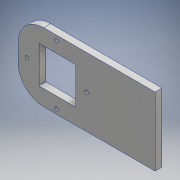
# Autodesk Inventor part: sholder_1
Saved by Autodesk Inventor 2016 (Build 200138000, 138)
## iProperties
Created: 2016-06-28
Part Number: sholder_1
Material: アルミニウム 6061
Document SubType Name: Modeling
Designer: 宏太
Density: 2.7 g/cm^3
Appearance: アルミニウム - フラット
Mass: 227.001 g
Surface Area: 264.508 cm^2
Volume: 84.0744 cm^3
Author: 宏太
Autodesk Inventor part; units mm, degrees
ref_plane "YZ Plane" through (0, 0, 0) normal (1, 0, 0) x (0, 1, 0)
ref_plane "XZ Plane" through (0, 0, 0) normal (0, 1, 0) x (-1, 0, 0)
ref_plane "XY Plane" through (0, 0, 0) normal (0, 0, 1) x (1, 0, 0)
sketch "スケッチ1" plane through (0, 0, 0) normal (0, 1, 0) x (-1, 0, 0)
  line L0 (-80, -40) -> (80, -40)
  line L1 (80, -40) -> (80, 40)
  line L2 (80, 40) -> (-80, 40)
  line L3 (-80, 40) -> (-80, -40)
  line L4 (-80, -40) -> (80, 40) construction
  line L5 (80, -40) -> (-80, 40) construction
  point P0 (0, 0)
  dimension "d0" = 160
  dimension "d1" = 80
  constraints: 12 end point, 2 midpoint, 2 parallel, 1 horizontal, 1 perpendicular
  measures "d0" distance of L2.end L1.end
  measures "d1" distance of L1.end L0.end
extrude "押し出し1" add sketch "スケッチ1" along normal blind 8
sketch "スケッチ2" plane through (0, 8, 0) normal (0, 1, 0) x (1, 0, 0)
  line L0 (-12.5, 21.5) -> (-55.5, 21.5)
  line L1 (-55.5, 21.5) -> (-55.5, -21.5)
  line L2 (-55.5, -21.5) -> (-12.5, -21.5)
  line L3 (-12.5, -21.5) -> (-12.5, 21.5)
  line L4 (-12.5, 21.5) -> (-55.5, -21.5) construction
  line L5 (-55.5, 21.5) -> (-12.5, -21.5) construction
  line L6 (-80, 40) -> (-80, -40) projected
  line L7 (-80, -40) -> (80, -40) projected
  point P0 (0, 0)
  point P1 (-34, 0)
  dimension "d4" = 43
  dimension "d5" = 43
  dimension "d20" = 46
  dimension "d21" = 40
  constraints: 12 end point, 2 midpoint, 2 parallel, 1 horizontal, 1 perpendicular
  measures "d4" distance of L2.end L1.end
  measures "d5" distance of L1.end L0.end
  measures "d20" distance from line of L6 point (-34, 0)
  measures "d21" distance from line of L7 point (-34, 0)
extrude "押し出し2" cut sketch "スケッチ2" against normal blind 8
sketch "スケッチ3" plane through (0, 8, 0) normal (0, 1, 0) x (1, 0, 0)
  circle A0 centre (-35, 0) radius 34.5
  circle A1 centre (-69.5, 0) radius 2.1
  circle A2 centre (-35, 34.5) radius 2.1
  circle A3 centre (0, 0) radius 2.1
  circle A4 centre (-35, -34.5) radius 2.1
  dimension "d8" = 69
  dimension "d9" = 35
  dimension "d10" = 4.2
  dimension "d11" = 4.2
  dimension "d12" = 4.2
  dimension "d13" = 4.2
  constraints: 5 centre point, 3 point on circle, 1 coincident
  measures "d8" diameter of A0
  measures "d9" distance of point (0, 0) A0.centre
  measures "d10" diameter of A1
  measures "d11" diameter of A2
  measures "d12" diameter of A3
  measures "d13" diameter of A4
extrude "押し出し3" cut sketch "スケッチ3" against normal blind 8 contours A0 A3 | A0 A3 | A2 A0 | A0 A2 | A4 A0 | A0 A4 | A1 A0 | A0 A1
fillet "フィレット1" radius 30 1 edges at (-80, 4, 40)
fillet "フィレット2" radius 30 1 edges at (-80, 4, -40)
